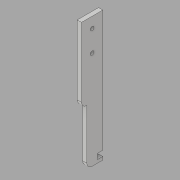
# Autodesk Inventor part: g_griper left jaw_arm
Saved by Autodesk Inventor 2019 (Build 230136000, 136)
## iProperties
Created: 2021-11-02
Part Number: g_griper left jaw_arm
Material: Generic
Document SubType Name: Modeling
Designer: Mohamed
Density: 1 g/cm^3
Appearance: Default
Author: Mohamed
Autodesk Inventor part; units mm, degrees
ref_plane "YZ Plane" through (0, 0, 0) normal (1, 0, 0) x (0, 1, 0)
ref_plane "XZ Plane" through (0, 0, 0) normal (0, 1, 0) x (-1, 0, 0)
ref_plane "XY Plane" through (0, 0, 0) normal (0, 0, 1) x (1, 0, 0)
sketch "Sketch1" plane through (0, 0, 0) normal (1, 0, 0) x (0, 1, 0)
  line L0 (5, 0) -> (70, 0)
  line L1 (70, 0) -> (70, -20)
  line L2 (70, -20) -> (0, -20)
  line L3 (0, -5) -> (0, -5)
  circle A0 centre (60, -10) radius 1.75
  circle A1 centre (40, -10) radius 1.75
  line L4 (0, -20) -> (-45, -20)
  line L5 (-45, -20) -> (-45, -10)
  line L6 (-40, -5) -> (0, -5)
  arc A2 (5, 0) -> (0, -5) centre (5, -5) ccw
  arc A3 (-40, -5) -> (-45, -10) centre (-40, -10) ccw
  point P0 (0, 0)
  point P1 (-45, -5)
  dimension "d0" = 70
  dimension "d1" = 20
  dimension "d4" = 3.5
  dimension "d5" = 3.5
  dimension "d6" = 45
  dimension "d7" = 15
  dimension "d8" = 5
  constraints: 14 end point, 4 centre point, 4 point on circle, 4 point on line, 4 tangent, 3 parallel, 2 horizontal, 2 perpendicular, 1 equal radius
  measures "d0" distance of L1.end L2.end
  measures "d1" distance of L0.end L1.end
  measures "d4" diameter of A0
  measures "d5" diameter of A1
  measures "d6" distance of L3.start point (-45, -5)
  measures "d7" distance of L4.end point (-45, -5)
  measures "d8" radius of A2
extrude "Extrusion1" add sketch "Sketch1" along normal blind 4
sketch "Sketch2" plane through (4, 0, 0) normal (1, 0, 0) x (0, 0, -1)
  arc A0 (5, -40) -> (10, -45) centre (10, -40) ccw projected
  line L0 (20, -52) -> (10, -52)
  line L1 (5, -47) -> (5, -40)
  arc A1 (5, -47) -> (10, -52) centre (10, -47) ccw
  line L2 (20, -52) -> (20, -49)
  line L3 (20, -49) -> (15, -49)
  line L4 (15, -49) -> (15, -39)
  line L5 (15, -39) -> (20, -39)
  line L6 (5, -40) -> (15, -40)
  point P0 (0, 0)
  point P1 (5, -52)
  dimension "d11" = 15
  dimension "d13" = 5
  dimension "d14" = 3
  dimension "d15" = 5
  dimension "d16" = 10
  constraints: 14 end point, 4 perpendicular, 4 point on line, 2 point on circle, 2 tangent, 1 centre point, 1 vertical
  measures "d11" distance of L0.start point (5, -52)
  measures "d13" radius of A1
  measures "d14" distance of L0.start L2.end
  measures "d15" distance of L2.end L3.end
  measures "d16" distance of L3.end L4.end
extrude "Extrusion2" add sketch "Sketch2" against normal blind 4
sketch "Sketch3" plane through (4, 0, 0) normal (1, 0, 0) x (0, 0, -1)
  line L0 (15, -45) -> (20, -45) projected
  line L1 (15, -45) -> (20, -45)
  line L2 (20, -45) -> (20, -44)
  line L3 (20, -44) -> (15, -44)
  line L4 (15, -44) -> (15, -45)
  point P0 (0, 0)
  dimension "d19" = 5
  dimension "d20" = 1
  constraints: 8 end point, 2 parallel, 1 horizontal, 1 perpendicular
  measures "d19" distance of L3.end L2.end
  measures "d20" distance of L2.end L1.end
extrude "Extrusion3" cut sketch "Sketch3" against normal blind 4
body "Solid1"
